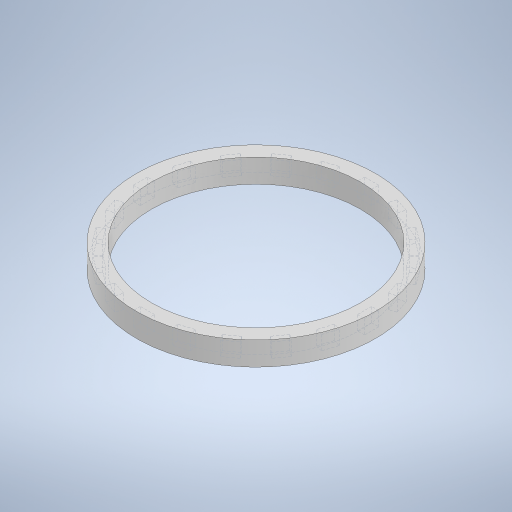
# Autodesk Inventor part: ring_ABS
Saved by Autodesk Inventor 2023 (Build 270158000, 158)
## iProperties
Created: 2023-07-04
Part Number: ring_ABS
Material: Generic
Document SubType Name: Modeling
Designer: checo
Density: 1 g/cm^3
Appearance: Default
Author: checo
Autodesk Inventor part; units mm, degrees
ref_plane "YZ Plane" through (0, 0, 0) normal (1, 0, 0) x (0, 1, 0)
ref_plane "XZ Plane" through (0, 0, 0) normal (0, 1, 0) x (-1, 0, 0)
ref_plane "XY Plane" through (0, 0, 0) normal (0, 0, 1) x (1, 0, 0)
sketch "Sketch1" plane through (0, 0, 0) normal (0, 1, 0) x (-1, 0, 0)
  circle A0 centre (0, 0) radius 50.8
  circle A1 centre (0, 0) radius 44.45
  dimension "d0" = 88.9
  dimension "d1" = 101.6
  constraints: 2 centre point, 2 coincident
  measures "d0" diameter of A1
  measures "d1" diameter of A0
extrude "Extrusion1" add sketch "Sketch1" along normal mid plane 10
sketch "Sketch2" plane through (0, 0, 0) normal (0, 1, 0) x (-1, 0, 0)
  circle A0 centre (0, 0) radius 50.8 construction
  line L0 (50.8, 0) -> (44.45, 0) construction
  circle A1 centre (0, 0) radius 44.45 construction
  line L1 (46.125, 3) -> (49.125, 3)
  line L2 (49.125, 3) -> (49.125, -3)
  line L3 (49.125, -3) -> (46.125, -3)
  line L4 (46.125, -3) -> (46.125, 3)
  line L5 (46.125, 3) -> (49.125, -3) construction
  line L6 (49.125, 3) -> (46.125, -3) construction
  line L7 (42.9404, -17.1066) -> (44.7945, -11.4002)
  line L8 (45.7936, -18.0336) -> (42.9404, -17.1066)
  line L9 (47.6477, -12.3273) -> (45.7936, -18.0336)
  line L10 (44.7945, -11.4002) -> (47.6477, -12.3273)
  line L11 (35.5526, -29.5386) -> (39.0793, -24.6845)
  line L12 (37.9796, -31.302) -> (35.5526, -29.5386)
  line L13 (41.5063, -26.4479) -> (37.9796, -31.302)
  line L14 (39.0793, -24.6845) -> (41.5063, -26.4479)
  line L15 (24.6845, -39.0793) -> (29.5386, -35.5526)
  line L16 (26.4479, -41.5063) -> (24.6845, -39.0793)
  line L17 (31.302, -37.9796) -> (26.4479, -41.5063)
  line L18 (29.5386, -35.5526) -> (31.302, -37.9796)
  line L19 (11.4002, -44.7945) -> (17.1066, -42.9404)
  line L20 (12.3273, -47.6477) -> (11.4002, -44.7945)
  line L21 (18.0336, -45.7936) -> (12.3273, -47.6477)
  line L22 (17.1066, -42.9404) -> (18.0336, -45.7936)
  line L23 (-3, -46.125) -> (3, -46.125)
  line L24 (-3, -49.125) -> (-3, -46.125)
  line L25 (3, -49.125) -> (-3, -49.125)
  line L26 (3, -46.125) -> (3, -49.125)
  line L27 (-17.1066, -42.9404) -> (-11.4002, -44.7945)
  line L28 (-18.0336, -45.7936) -> (-17.1066, -42.9404)
  line L29 (-12.3273, -47.6477) -> (-18.0336, -45.7936)
  line L30 (-11.4002, -44.7945) -> (-12.3273, -47.6477)
  line L31 (-29.5386, -35.5526) -> (-24.6845, -39.0793)
  line L32 (-31.302, -37.9796) -> (-29.5386, -35.5526)
  line L33 (-26.4479, -41.5063) -> (-31.302, -37.9796)
  line L34 (-24.6845, -39.0793) -> (-26.4479, -41.5063)
  line L35 (-39.0793, -24.6845) -> (-35.5526, -29.5386)
  line L36 (-41.5063, -26.4479) -> (-39.0793, -24.6845)
  line L37 (-37.9796, -31.302) -> (-41.5063, -26.4479)
  line L38 (-35.5526, -29.5386) -> (-37.9796, -31.302)
  line L39 (-44.7945, -11.4002) -> (-42.9404, -17.1066)
  line L40 (-47.6477, -12.3273) -> (-44.7945, -11.4002)
  line L41 (-45.7936, -18.0336) -> (-47.6477, -12.3273)
  line L42 (-42.9404, -17.1066) -> (-45.7936, -18.0336)
  line L43 (-46.125, 3) -> (-46.125, -3)
  line L44 (-49.125, 3) -> (-46.125, 3)
  line L45 (-49.125, -3) -> (-49.125, 3)
  line L46 (-46.125, -3) -> (-49.125, -3)
  line L47 (-42.9404, 17.1066) -> (-44.7945, 11.4002)
  line L48 (-45.7936, 18.0336) -> (-42.9404, 17.1066)
  line L49 (-47.6477, 12.3273) -> (-45.7936, 18.0336)
  line L50 (-44.7945, 11.4002) -> (-47.6477, 12.3273)
  line L51 (-35.5526, 29.5386) -> (-39.0793, 24.6845)
  line L52 (-37.9796, 31.302) -> (-35.5526, 29.5386)
  line L53 (-41.5063, 26.4479) -> (-37.9796, 31.302)
  line L54 (-39.0793, 24.6845) -> (-41.5063, 26.4479)
  line L55 (-24.6845, 39.0793) -> (-29.5386, 35.5526)
  line L56 (-26.4479, 41.5063) -> (-24.6845, 39.0793)
  line L57 (-31.302, 37.9796) -> (-26.4479, 41.5063)
  line L58 (-29.5386, 35.5526) -> (-31.302, 37.9796)
  line L59 (-11.4002, 44.7945) -> (-17.1066, 42.9404)
  line L60 (-12.3273, 47.6477) -> (-11.4002, 44.7945)
  line L61 (-18.0336, 45.7936) -> (-12.3273, 47.6477)
  line L62 (-17.1066, 42.9404) -> (-18.0336, 45.7936)
  line L63 (3, 46.125) -> (-3, 46.125)
  line L64 (3, 49.125) -> (3, 46.125)
  line L65 (-3, 49.125) -> (3, 49.125)
  line L66 (-3, 46.125) -> (-3, 49.125)
  line L67 (17.1066, 42.9404) -> (11.4002, 44.7945)
  line L68 (18.0336, 45.7936) -> (17.1066, 42.9404)
  line L69 (12.3273, 47.6477) -> (18.0336, 45.7936)
  line L70 (11.4002, 44.7945) -> (12.3273, 47.6477)
  line L71 (29.5386, 35.5526) -> (24.6845, 39.0793)
  line L72 (31.302, 37.9796) -> (29.5386, 35.5526)
  line L73 (26.4479, 41.5063) -> (31.302, 37.9796)
  line L74 (24.6845, 39.0793) -> (26.4479, 41.5063)
  line L75 (39.0793, 24.6845) -> (35.5526, 29.5386)
  line L76 (41.5063, 26.4479) -> (39.0793, 24.6845)
  line L77 (37.9796, 31.302) -> (41.5063, 26.4479)
  line L78 (35.5526, 29.5386) -> (37.9796, 31.302)
  line L79 (44.7945, 11.4002) -> (42.9404, 17.1066)
  line L80 (47.6477, 12.3273) -> (44.7945, 11.4002)
  line L81 (45.7936, 18.0336) -> (47.6477, 12.3273)
  line L82 (42.9404, 17.1066) -> (45.7936, 18.0336)
  point P0 (47.625, 0)
  dimension "d4" = 3
  dimension "d5" = 6
  dimension "d8" = 360
  constraints: 166 end point, 3 midpoint, 2 coincident, 2 horizontal, 2 horizontal alignment, 2 parallel, 1 perpendicular, 1 point on line, 181 other
  measures "d4" distance of L2.end L3.end
  measures "d5" distance of L1.end L2.end
extrude "Extrusion2" cut sketch "Sketch2" along normal mid plane 6
body "Solid1"
